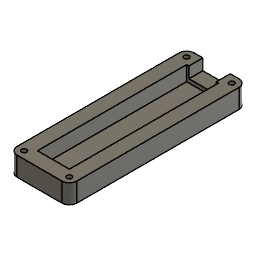
Body (Autodesk Fusion 360 design; units mm, degrees)
part number: 2026-01-31-17-47-11-439
Autodesk Fusion 360 part; units mm, degrees
sketch "Sketch1" plane through (0, 0, 0) normal (0, 1, 0) x (1, 0, 0)
  line L0 (0, 0) -> (21.6, 0)
  line L1 (21.6, 0) -> (21.6, -101)
  line L2 (21.6, -101) -> (0, -101)
  line L3 (0, -101) -> (0, 0)
  line L4 (-9.5, 9.5) -> (31.1, 9.5)
  line L5 (31.1, 9.5) -> (31.1, -110.5)
  line L6 (31.1, -110.5) -> (-9.5, -110.5)
  line L7 (-9.5, -110.5) -> (-9.5, 9.5)
  circle A0 centre (-4.5, -105.5) radius 1.7
  circle A1 centre (26.1, -105.5) radius 1.7
  circle A2 centre (26.1, 4.5) radius 1.7
  circle A3 centre (-4.5, 4.5) radius 1.7
  circle A4 centre (-4.5, 4.5) radius 3
  circle A5 centre (26.1, 4.5) radius 3
  circle A6 centre (26.1, -105.5) radius 3
  circle A7 centre (-4.5, -105.5) radius 3
  dimension "d1" = 21.6
  dimension "d2" = 101
  dimension "d3" = 40.6
  dimension "d4" = 120
  dimension "d5" = 9.5
  dimension "d6" = 9.5
  dimension "d7" = 3.4
  dimension "d8" = 3.4
  dimension "d9" = 3.4
  dimension "d10" = 3.4
  dimension "d11" = 5
  dimension "d12" = 5
  dimension "d13" = 5
  dimension "d14" = 5
  dimension "d15" = 5
  dimension "d16" = 5
  dimension "d17" = 5
  dimension "d18" = 5
  dimension "d19" = 6
  dimension "d20" = 6
  dimension "d21" = 6
  dimension "d22" = 6
  constraint horizontal L0
  constraint vertical L1
  constraint horizontal L2
  constraint vertical L3
  constraint coincident L0.start L3.end
  constraint horizontal L4
  constraint vertical L5
  constraint horizontal L6
  constraint vertical L7
  constraint concentric A3 A4
  constraint concentric A2 A5
  constraint concentric A1 A6
  constraint concentric A0 A7
  measures "d1" distance of L0.start L0.end
  measures "d2" distance of L0.start L2.end
  measures "d3" distance of L4.start L4.end
  measures "d4" distance of L4.start L6.end
  measures "d5" distance of L3 L7
  measures "d6" distance of L0 L4
  measures "d7" diameter of A0
  measures "d8" diameter of A1
  measures "d9" diameter of A2
  measures "d10" diameter of A3
  measures "d11" distance of L4 A2.centre
  measures "d12" distance of L5 A2.centre
  measures "d13" distance of L6 A1.centre
  measures "d14" distance of L5 A1.centre
  measures "d15" distance of L6 A0.centre
  measures "d16" distance of L7 A0.centre
  measures "d17" distance of L4 A3.centre
  measures "d18" distance of L7 A3.centre
  measures "d19" diameter of A4
  measures "d20" diameter of A5
  measures "d21" diameter of A6
  measures "d22" diameter of A7
extrude "Extrude1" add sketch "Sketch1" along normal blind 9.9 from surface at 3.1 contours A4 | A5 | A6 | A7 makes body 1 at (29.0963, 9.7, -4.3505) makes body 2 at (-1.5037, 9.7, -4.3505) makes body 3 at (28.6599, 9.7, 103.9357) makes body 4 at (-7.2644, 9.7, 106.6653)
extrude "Extrude2" add sketch "Sketch1" along normal blind 13 contours L4 L5 L6 L7 bodies 1 2 3 4
extrude "Extrude3" add sketch "Sketch1" along normal blind 3 contours L0 L1 L2 L3 bodies 1
sketch "Sketch2" plane through (0, 13, 0) normal (0, 1, 0) x (-1, 0, 0)
  circle A0 centre (-26.1, -4.5) radius 1.7
  circle A1 centre (4.5, 105.5) radius 1.7
  line L0 (-21.6, 101) -> (0, 101)
  line L1 (0, 101) -> (0, 0)
  line L2 (0, 0) -> (-21.6, 0)
  line L3 (-21.6, 0) -> (-21.6, 101)
  line L4 (9.5, 110.5) -> (-31.1, 110.5)
  line L5 (-31.1, 110.5) -> (-31.1, -9.5)
  line L6 (-31.1, -9.5) -> (9.5, -9.5)
  line L7 (9.5, -9.5) -> (9.5, 110.5)
  circle A2 centre (4.5, -4.5) radius 1.7
  circle A3 centre (-26.1, 105.5) radius 1.7
  line L8 (-1.55, -9.5) -> (-20.05, -9.5)
  line L9 (-20.05, -9.5) -> (-20.05, 0)
  line L10 (-20.05, 0) -> (-1.55, 0)
  line L11 (-1.55, 0) -> (-1.55, -9.5)
  dimension "d30" = 11.05
  dimension "d31" = 18.5
  constraint horizontal L8
  constraint vertical L9
  constraint horizontal L10
  constraint vertical L11
  measures "d30" distance of L6.end L8.start
  measures "d31" distance of L8.start L8.end
extrude "Extrude4" cut sketch "Sketch2" against normal blind 7.5 contours L2 L6 L8 L9 L10 L11 bodies 1
fillet "Fillet1" radius 5 4 edges at (31.1, 6.5, -9.5) (-9.5, 6.5, -9.5) (-9.5, 6.5, 110.5) (31.1, 6.5, 110.5) on bodies 1
